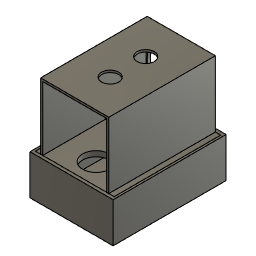
Bloc mesure v17 (Autodesk Fusion 360 design; units mm, degrees)
Autodesk Fusion 360 part; units mm, degrees
sketch "Esquisse1" plane through (0, 0, 0) normal (0, 0, 1) x (1, 0, 0)
  line L0 (0, 0) -> (60, 0)
  line L1 (60, 0) -> (60, 60)
  line L2 (60, 60) -> (0, 60)
  line L3 (0, 60) -> (0, 0)
  line L4 (-2, -3) -> (62, -3)
  line L5 (62, -3) -> (62, 62)
  line L6 (62, 62) -> (-2, 62)
  line L7 (-2, 62) -> (-2, -3)
  circle A0 centre (30, 30) radius 29
  circle A1 centre (5, 55) radius 2
  circle A2 centre (55, 55) radius 2
  circle A3 centre (5, 5) radius 2
  circle A4 centre (55, 5) radius 2
  line L8 (0, 0) -> (0, -3)
  line L9 (60, 0) -> (60, -3)
  line L10 (0, 0) -> (-2, 0)
  line L11 (60, 0) -> (62, 0)
  line L12 (-2, 0) -> (-7, 0)
  line L13 (-7, 0) -> (-7, -5)
  line L14 (-7, -5) -> (67, -5)
  line L15 (67, -5) -> (67, 0)
  line L16 (67, 0) -> (62, 0)
  line L17 (-7, 0) -> (-9, 0)
  line L18 (-9, 0) -> (-9, -37.428)
  line L19 (-9, -37.428) -> (69, -37.428)
  line L20 (69, -37.428) -> (69, 0)
  line L21 (69, 0) -> (67, 0)
  line L22 (-7, -5) -> (-3.362, -5)
  line L23 (-4, -5) -> (-4, -34.428)
  line L24 (-4, -34.428) -> (64, -34.428)
  line L25 (64, -34.428) -> (64, -5)
  line L26 (64, -5) -> (67, -5)
  dimension "d1" = 60
  dimension "d2" = 60
  dimension "d3" = 2
  dimension "d4" = 2
  dimension "d5" = 2
  dimension "d6" = 3
  dimension "d7" = 58
  dimension "d8" = 30
  dimension "d9" = 30
  dimension "d10" = 4
  dimension "d11" = 4
  dimension "d12" = 4
  dimension "d13" = 4
  dimension "d14" = 5
  dimension "d15" = 5
  dimension "d16" = 5
  dimension "d17" = 5
  dimension "d18" = 5
  dimension "d19" = 5
  dimension "d20" = 5
  dimension "d21" = 5
  dimension "d51" = 5
  dimension "d52" = 5
  dimension "d53" = 2
  dimension "d56" = 2
  dimension "d57" = 2
  dimension "d58" = 5
  dimension "d59" = 3
  dimension "d60" = 5
  constraint horizontal L0
  constraint vertical L1
  constraint horizontal L2
  constraint vertical L3
  constraint coincident L0.start L3.end
  constraint horizontal L4
  constraint vertical L5
  constraint horizontal L6
  constraint vertical L7
  constraint coincident L4 L8.end
  constraint perpendicular L4 L8
  constraint coincident L4 L9.end
  constraint perpendicular L4 L9
  constraint coincident L7 L10.end
  constraint perpendicular L7 L10
  constraint coincident L5 L11.end
  constraint perpendicular L5 L11
  constraint perpendicular L7 L12
  constraint perpendicular L12 L13
  constraint perpendicular L7 L14
  constraint perpendicular L14 L15
  constraint perpendicular L5 L16
  constraint perpendicular L13 L17
  constraint perpendicular L17 L18
  constraint perpendicular L13 L19
  constraint perpendicular L19 L20
  constraint perpendicular L15 L21
  constraint coincident L14 L22.end
  constraint coincident L14 L23.start
  constraint perpendicular L14 L23
  constraint perpendicular L23 L24
  constraint perpendicular L24 L25
  constraint perpendicular L15 L26
  measures "d1" distance of L1.end L2.end
  measures "d2" distance of L0.end L1.end
  measures "d3" distance of L3 L7
  measures "d4" distance of L1 L5
  measures "d5" distance of L2 L6
  measures "d6" distance of L0 L4
  measures "d7" diameter of A0
  measures "d8" distance of L3 A0.centre
  measures "d9" distance of L2 A0.centre
  measures "d10" diameter of A1
  measures "d11" diameter of A2
  measures "d12" diameter of A3
  measures "d13" diameter of A4
  measures "d14" distance of L3 A1.centre
  measures "d15" distance of L2 A1.centre
  measures "d16" distance of L2 A2.centre
  measures "d17" distance of L1 A2.centre
  measures "d18" distance of L0 A3.centre
  measures "d19" distance of L3 A3.centre
  measures "d20" distance of L1 A4.centre
  measures "d21" distance of L0 A4.centre
  measures "d51" distance of L7 L13
  measures "d52" distance of L5 L15
  measures "d53" distance of L4 L14
  measures "d56" distance of L13 L18
  measures "d57" distance of L15 L20
  measures "d58" distance of L20 L25
  measures "d59" distance of L19 L24
  measures "d60" distance of L18 L23
extrude "Extrusion1" add sketch "Esquisse1" along normal blind 3 contours L0 L1 L2 L3 makes body 1
extrude "Extrusion2" add sketch "Esquisse1" along normal blind 100 and the other way blind 0 contours L1 L2 L3 L5 L6 L7 L10 L11 | L4 L7 L8 L10 | L4 L5 L9 L11 bodies 1
sketch "Esquisse3" plane through (0, 60, 0) normal (0, -1, 0) x (1, 0, 0)
  line L0 (0, 3) -> (60, 3)
  line L1 (60, 3) -> (60, 100)
  line L2 (60, 100) -> (0, 100)
  line L3 (0, 100) -> (0, 3)
  line L4 (44.0145, 78.9655) -> (49.4524, 81.5012)
  line L5 (49.4524, 81.5012) -> (41, 99.6274)
  line L6 (41, 99.6274) -> (35.5622, 97.0917)
  line L7 (35.5622, 97.0917) -> (44.0145, 78.9655)
  dimension "d37" = 20
  dimension "d38" = 6
  dimension "d39" = 25
  dimension "d40" = 19
  constraint perpendicular L4 L5
  constraint parallel L4 L6
  constraint parallel L5 L7
  measures "d37" distance of L4.end L5.end
  measures "d38" distance of L5.end L6.end
  measures "d39" angle of L1 L5
  measures "d40" distance of L1 L5.end
extrude "Extrusion5" add sketch "Esquisse1" along normal blind 100 and the other way blind 0 separate body contours L0 L4 L8 L9 | L4 L5 L7 L12 L13 L14 L15 L16 L22 L26 makes body 2
extrude "Extrusion6" add sketch "Esquisse1" along normal blind 100 and the other way blind 0 separate body contours L13 L14 L15 L17 L18 L19 L20 L21 L22 L23 L24 L25 L26 makes body 3
sketch "Esquisse4" plane through (0, 0, 0) normal (0, 1, 0) x (-1, 0, 0)
  line L0 (0, 0) -> (0, 100)
  line L1 (0, 100) -> (-60, 100)
  line L2 (-60, 100) -> (-60, 0)
  line L3 (-60, 0) -> (0, 0)
  circle A0 centre (-30, 33.4) radius 4
  circle A1 centre (-30, 80) radius 12.55
  dimension "d90" = 8
  dimension "d91" = 25.1
  dimension "d92" = 20
  dimension "d93" = 30
  dimension "d94" = 30
  dimension "d95" = 66.6
  measures "d90" diameter of A0
  measures "d91" diameter of A1
  measures "d92" distance of L1 A1.centre
  measures "d93" distance of L0 A1.centre
  measures "d94" distance of L0 A0.centre
  measures "d95" distance of L1 A0.centre
sketch "Esquisse5" plane through (0, 62, 0) normal (0, 1, 0) x (-1, 0, 0)
  line L0 (2, 0) -> (2, 100)
  line L1 (2, 100) -> (-62, 100)
  line L2 (-62, 100) -> (-62, 0)
  line L3 (-62, 0) -> (2, 0)
  circle A0 centre (-30, 33.4) radius 8.05
  line L4 (0, 0) -> (0, 100)
  circle A1 centre (-30, 66.7) radius 8.05
  dimension "d81" = 16.1
  dimension "d83" = 30
  dimension "d84" = 66.6
  dimension "d85" = 16.1
  dimension "d86" = 30
  dimension "d87" = 33.3
  measures "d81" diameter of A0
  measures "d83" distance of A0.centre L4
  measures "d84" distance of L1 A0.centre
  measures "d85" diameter of A1
  measures "d86" distance of L4 A1.centre
  measures "d87" distance of L1 A1.centre
extrude "Extrusion11" cut sketch "Esquisse5" against normal blind 5 contours A0 | A1 bodies 1
extrude "Extrusion12" cut sketch "Esquisse4" against normal blind 5 contours A0 | A1 bodies 2
extrude "Extrusion13" add sketch "Esquisse1" against normal blind 3 contours L0 L4 L8 L9 | L4 L7 L8 L10 | L4 L5 L9 L11 | L4 L5 L7 L12 L13 L14 L15 L16 L22 L26 | L13 L14 L15 L17 L18 L19 L20 L21 L22 L23 L24 L25 L26 | L14 L22 L23 L24 L25 bodies 3
extrude "Extrusion14" add sketch "Esquisse1" along normal blind 3 from surface at 100 contours L0 L4 L8 L9 | L4 L7 L8 L10 | L4 L5 L9 L11 | L4 L5 L7 L12 L13 L14 L15 L16 L22 L26 | L13 L14 L15 L17 L18 L19 L20 L21 L22 L23 L24 L25 L26 | L14 L22 L23 L24 L25 bodies 3
